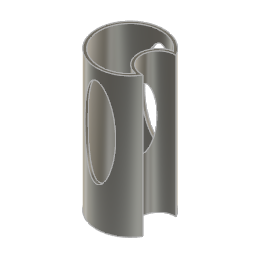
usb-guidance v1 (Autodesk Fusion 360 design; units mm, degrees)
Autodesk Fusion 360 part; units mm, degrees
note: some values were not read from the file. Set by a fixed rule: which sketch regions a step uses.
sketch "Sketch1" plane through (0, 0, 0) normal (0, 0, 1) x (1, 0, 0)
  circle A0 centre (0, 0) radius 6
  circle A1 centre (0, 0) radius 5.5
  circle A2 centre (4.9955, 0.0458) radius 3
  circle A3 centre (4.9955, 0.0458) radius 3.5
  dimension "d1" = 12
  dimension "d2" = 11
  dimension "d4" = 6
  dimension "d5" = 7
  constraint coincident A0.centre A1.centre
  constraint concentric A2 A3
  measures "d1" diameter of A0
  measures "d2" diameter of A1
  measures "d4" diameter of A2
  measures "d5" diameter of A3
extrude "Extrude1" add sketch "Sketch1" along normal blind 25 contours A0 A1 A2 A3 | A0 A1 A2 A3 | A0 A1 A3 | A1 A2 A3
ref_plane "WorkPlane1" through (0, -6, 10.4032) normal (0, -1, 0) x (-1, 0, 0)
sketch "Sketch2" plane through (0, -6, 0) normal (0, -1, 0) x (-1, 0, 0)
  ellipse E0 centre (0, -15) end of major axis (0, -23) minor radius 2.75
  line L0 (0, -7) -> (0, -23) construction
  line L1 (-2.75, -15) -> (2.75, -15) construction
  dimension "d9" = 5.5
  constraint coincident E0 L0.start
  constraint coincident E0 L0.end
  constraint coincident E0 L1.start
  constraint coincident E0 L1.end
  constraint vertical L0
extrude "Extrude2" cut sketch "Sketch2" against normal blind 20
sketch "Sketch3" plane through (0, 0, 0) normal (0, 0, 1) x (1, 0, 0)
  line L0 (-63, 9) -> (-37, 9)
  line L1 (-37, 9) -> (-37, -12)
  line L2 (-37, -12) -> (-63, -12)
  line L3 (-63, -12) -> (-63, 9)
  constraint horizontal L0
  constraint vertical L1
  constraint horizontal L2
  constraint vertical L3
extrude "Extrude3" [suppressed]
sketch "Sketch4" plane through (0, -12, 0) normal (0, -1, 0) x (1, 0, 0)
  line L0 (-63, 0) -> (-37, 0)
  line L1 (-37, 0) -> (-37, 47)
  line L2 (-37, 47) -> (-63, 47)
  line L3 (-63, 47) -> (-63, 0)
  circle A0 centre (-54, 23) radius 2
  circle A1 centre (-54, 32) radius 2
  dimension "d14" = 4
  dimension "d15" = 4
  dimension "d16" = 9
  dimension "d17" = 15
  dimension "d18" = 23
  measures "d14" diameter of A0
  measures "d15" diameter of A1
  measures "d16" distance of A0.centre A1.centre
  measures "d17" distance of L2 A1.centre
  measures "d18" distance of L0 A0.centre
equation "d2 = d1 - 1 mm"
